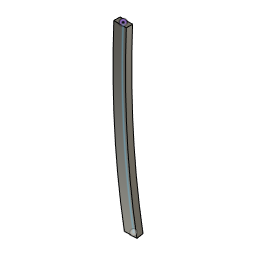
Propellergondel (Autodesk Fusion 360 archive; units mm, degrees)
design "Boom"
Autodesk Fusion 360 part; units mm, degrees
sketch "Skizze1" plane through (0, 0, 0) normal (0, 0, 1) x (1, 0, 0)
  line L0 (5, 2.5) -> (-5, 2.5)
  line L1 (-5, 2.5) -> (-5, -2.5)
  line L2 (-5, -2.5) -> (5, -2.5)
  line L3 (5, -2.5) -> (5, 2.5)
  line L4 (5, 2.5) -> (-5, -2.5) construction
  line L5 (-5, 2.5) -> (5, -2.5) construction
  dimension "d1" = 10
  dimension "d2" = 5
  constraint horizontal L0
  constraint perpendicular L0 L1
  constraint parallel L0 L2
  constraint parallel L1 L3
  constraint coincident L4 origin
  constraint coincident L5 origin
  measures "d1" distance of L1.end L2.end
  measures "d2" distance of L0.end L1.end
sketch "Skizze2" plane through (0, 0, 0) normal (1, 0, 0) x (0, 1, 0)
  arc A0 (0, 0) -> (8.4117, -149.7359) centre (781.2358, -31.2166) ccw
  constraint coincident A0.start origin
sweep "Sweeping1" add profiles "Skizze1" path "Skizze2" along A0 section 1

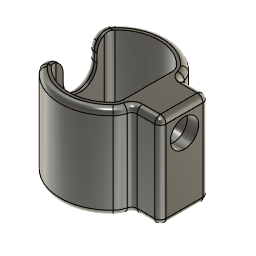
design "TVC"
Autodesk Fusion 360 part; units mm, degrees
sketch "Skizze1" plane through (0, 0, 0) normal (0, 0, 1) x (1, 0, 0)
  line L0 (0, 0) -> (0, 16)
  line L1 (0, 16) -> (12, 16) construction
  line L2 (12, 16) -> (12, 0)
  line L3 (12, 0) -> (0, 0) construction
  line L4 (12, 8) -> (12, 12.2749) construction
  line L5 (12, 8) -> (12, 3.7251) construction
  line L6 (0, 8) -> (0, 12.2749) construction
  line L7 (0, 8) -> (0, 3.7251) construction
  arc A0 (11.4545, 13.6476) -> (0.5455, 13.6476) centre (6, 8.5) ccw
  arc A1 (0.5455, 2.3524) -> (11.4545, 2.3524) centre (6, 7.5) ccw
  arc A2 (0.5455, 13.6476) -> (0, 12.2749) centre (2, 12.2749) ccw
  arc A3 (12, 12.2749) -> (11.4545, 13.6476) centre (10, 12.2749) ccw
  arc A4 (0, 3.7251) -> (0.5455, 2.3524) centre (2, 3.7251) ccw
  arc A5 (11.4545, 2.3524) -> (12, 3.7251) centre (10, 3.7251) ccw
  arc A6 (-1.5, 3.7251) -> (-0.5455, 1.3229) centre (2, 3.7251) ccw
  arc A7 (-0.5455, 1.3229) -> (12.5455, 1.3229) centre (6, 7.5) ccw
  arc A8 (12.5455, 1.3229) -> (13.5, 3.7251) centre (10, 3.7251) ccw
  line L8 (13.5, 8) -> (13.5, 3.7251)
  line L9 (13.5, 8) -> (13.5, 12.2749)
  arc A9 (13.5, 12.2749) -> (12.5455, 14.6771) centre (10, 12.2749) ccw
  arc A10 (12.5455, 14.6771) -> (-0.5455, 14.6771) centre (6, 8.5) ccw
  arc A11 (-0.5455, 14.6771) -> (-1.5, 12.2749) centre (2, 12.2749) ccw
  line L10 (-1.5, 8) -> (-1.5, 12.2749)
  line L11 (-1.5, 8) -> (-1.5, 3.7251)
  line L12 (12, 8) -> (0, 8)
  circle A12 centre (6, 8) radius 3
  point P0 (12, 13)
  point P1 (12, 3)
  point P2 (0, 13)
  point P3 (0, 3)
  dimension "d1" = 16
  dimension "d2" = 12
  dimension "d3" = 16
  dimension "d4" = 5
  dimension "d5" = 5
  dimension "d6" = 5
  dimension "d7" = 5
  dimension "d8" = 2
  dimension "d9" = 2
  dimension "d10" = 2
  dimension "d11" = 2
  dimension "d12" = 1.5
  dimension "d15" = 6
  constraint coincident L0.start L3.end
  constraint vertical L0
  constraint perpendicular L0 L1
  constraint perpendicular L1 L2
  constraint midpoint L2 L4.start
  constraint perpendicular L3 L4
  constraint parallel L2 L5
  constraint midpoint L0 L6.start
  constraint parallel L0 L6
  constraint parallel L0 L7
  constraint tangent L1 A0
  constraint tangent L3 A1
  constraint coincident P2 L6
  constraint coincident P2 A0
  constraint tangent L6 A2
  constraint tangent A0 A2
  constraint coincident P0 L4
  constraint coincident P0 A0
  constraint tangent L4 A3
  constraint tangent A0 A3
  constraint coincident P3 L7
  constraint coincident P3 A1
  constraint tangent L7 A4
  constraint tangent A1 A4
  constraint coincident P1 L5
  constraint coincident P1 A1
  constraint tangent L5 A5
  constraint tangent A1 A5
  constraint midpoint L12 A12.centre
  measures "d1" distance of L0.start L0.end
  measures "d2" distance of L0.end L1.end
  measures "d3" distance of L1.end L2.end
  measures "d4" distance of L4.start P0
  measures "d5" distance of L4.start P1
  measures "d6" distance of L6.start P2
  measures "d7" distance of L6.start P3
  measures "d8" radius of A2
  measures "d9" radius of A3
  measures "d10" radius of A4
  measures "d11" radius of A5
  measures "d15" diameter of A12
extrude "Extrusion1" add sketch "Skizze1" along normal blind 5 contours L0 A6 A7 A10 A11 L10 L11 | L0 L2 A1 A4 A5 A7 | L0 L2 A0 A2 A3 A10
extrude "Extrusion2" add sketch "Skizze1" along normal blind 1.5 contours L0 L2 A1 A4 A5 L12 A12 | L0 L2 A0 A2 A3 L12 A12
extrude "Extrusion3" add sketch "Skizze1" along normal blind 25 contours L0 A6 A7 A10 A11 L10 L11 | L0 L2 A1 A4 A5 A7 | L0 L2 A0 A2 A3 A10 | L2 A7 A8 L8 L9 A9 A10
sketch "Skizze2" plane through (13.5, 0, 0) normal (1, 0, 0) x (0, 1, 0)
  line L0 (3.7251, 0) -> (12.2749, 0)
  line L1 (12.2749, 0) -> (12.2749, 25)
  line L2 (12.2749, 25) -> (3.7251, 25)
  line L3 (3.7251, 25) -> (3.7251, 0)
  line L4 (8, 25) -> (8, 12.5)
  circle A0 centre (8, 12.5) radius 2.5
  circle A1 centre (8, 12.5) radius 4
  dimension "d20" = 12.5
  dimension "d21" = 5
  dimension "d22" = 8
  constraint midpoint L2 L4.start
  constraint perpendicular L2 L4
  constraint coincident L4.end A0.centre
  measures "d20" distance of L4.start L4.end
  measures "d21" diameter of A0
  measures "d22" diameter of A1
extrude "Extrusion4" add sketch "Skizze2" along normal blind 5 contours A1
extrude "Extrusion5" add 1 faces at (13.5, 8.0996, 22.1629) along direction (1, 0, 0) blind 5
fillet "Abrundung1" radius 1 4 edges at (13.5, 3.7251, 12.5) (13.5, 12.2749, 12.5) (18.5, 12.2749, 12.5) (18.5, 3.7251, 12.5)
sketch "Skizze3" plane through (13.5, 0, 0) normal (1, 0, 0) x (0, 1, 0)
  circle A0 centre (8, 12.5) radius 2.5
  circle A1 centre (8, 12.5) radius 1.5
  dimension "d29" = 3
  constraint concentric A0 A1
  measures "d29" diameter of A1
extrude "Extrusion6" cut sketch "Skizze3" against normal blind 1.5 contours A1
sketch "Skizze4" plane through (-1.5, 0, 0) normal (-1, 0, 0) x (0, -1, 0)
  line L0 (-12.2749, 0) -> (-3.7251, 0)
  line L1 (-3.7251, 0) -> (-3.7251, 25)
  line L2 (-3.7251, 25) -> (-12.2749, 25)
  line L3 (-12.2749, 25) -> (-12.2749, 0)
  circle A0 centre (-8, 12.5) radius 1.5
  circle A1 centre (-8, 12.5) radius 4
  dimension "d32" = 8
  constraint concentric A0 A1
  measures "d32" diameter of A1
extrude "Extrusion7" [suppressed]
chamfer "Fase1" [suppressed]
extrude "Extrusion8" add 1 faces at (13.5, 10.1518, 12.6987) along direction (1, 0, 0) blind 1.5
chamfer "Fase2" distance 1.5 distance2 0.5 1 edges at (15, 5.6692, 13.404) measured on face at (16.1667, 10.4969, 12.6246)
sketch "Skizze5" plane through (12, 0, 0) normal (-1, 0, 0) x (0, -1, 0)
  circle A0 centre (-8, 12.5) radius 1.5
  line L0 (-12.2749, 1.5) -> (-3.7251, 1.5)
  line L1 (-3.7251, 1.5) -> (-3.7251, 25)
  line L2 (-3.7251, 25) -> (-12.2749, 25)
  line L3 (-12.2749, 25) -> (-12.2749, 1.5)
  circle A1 centre (-8, 12.5) radius 3
  dimension "d41" = 6
  constraint concentric A0 A1
  measures "d41" diameter of A1
extrude "Extrusion9" cut sketch "Skizze5" against normal blind 1 contours A1
extrude "Extrusion10" cut 1 faces at (13, 5.5168, 12.2764) along direction (1, 0, 0) blind 0.75
move_face "Flächen versetzen1" offset -8.5 1 faces at (15.7583, 6.9084, 25)
sketch "Skizze6" plane through (-1.5, 0, 0) normal (-1, 0, 0) x (0, -1, 0)
  line L0 (-12.2749, 0) -> (-3.7251, 0)
  line L1 (-3.7251, 0) -> (-3.7251, 16.5)
  line L2 (-3.7251, 16.5) -> (-12.2749, 16.5)
  line L3 (-12.2749, 16.5) -> (-12.2749, 0)
  circle A0 centre (-8, 12.5) radius 1.5
  circle A1 centre (-8, 12.5) radius 3
  line L4 (-8, 12.5) -> (-5, 12.5) construction
  line L5 (-8, 12.5) -> (-11, 12.5) construction
  line L6 (-5, 12.5) -> (-5, 16.5)
  line L7 (-11, 12.5) -> (-11, 16.5)
  constraint coincident A0.centre A1.centre
  constraint coincident A1 L4.end
  constraint parallel L2 L4
  constraint coincident A1 L5.end
  constraint parallel L4 L5
  constraint coincident L2 L6.end
  constraint tangent A1 L6
  constraint coincident L2 L7.end
  constraint tangent A1 L7
extrude "Extrusion11" cut sketch "Skizze6" against normal blind 1.5 contours L2 A1 L6 L7 | A1 | A0
fillet "Abrundung2" radius 2.5 2 edges at (-0.75, 11, 16.5) (-0.75, 5, 16.5)
move_face "Flächen versetzen2" offset 0.5 1 faces at (14.1667, 9.4981, 12.5748)
fillet "Abrundung3" radius 1 20 edges at (18.2071, 4.018, 16.5) (18.5, 8, 16.5) (18.2071, 11.982, 16.5) (15.9437, 12.2749, 16.5) (13.7639, 12.4932, 16.5) (13.0877, 13.923, 16.5) (6, 17.5, 16.5) (-0.9709, 14.1252, 16.5) (-1.4468, 12.8824, 16.4225) (-1.5, 11.3421, 15.2624) (-1.5, 11, 13.25) (-1.5, 8, 9.5) (-1.5, 5, 13.25) (-1.5, 4.6579, 15.2624) (-1.4468, 3.1176, 16.4225) (-0.9709, 1.8748, 16.5) (6, -1.5, 16.5) (13.0877, 2.077, 16.5) (13.7639, 3.5068, 16.5) (15.9437, 3.7251, 16.5)
fillet "Abrundung4" radius 1 14 edges at (-1.2526, 13.5674, 0) (6, 17.5, 0) (13.0877, 13.923, 0) (13.7639, 12.4932, 0) (15.9437, 12.2749, 0) (18.2071, 11.982, 0) (18.5, 8, 0) (18.2071, 4.018, 0) (15.9437, 3.7251, 0) (13.7639, 3.5068, 0) (13.0877, 2.077, 0) (6, -1.5, 0) (-1.2526, 2.4326, 0) (-1.5, 8, 0) 1 faces at (12.4923, 8, 0)
named bodies: "tvc"
